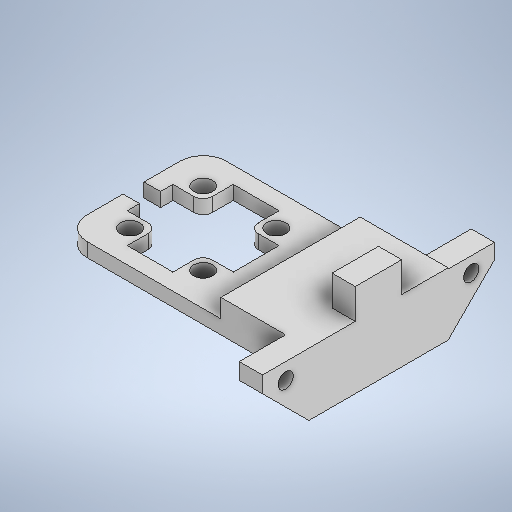
# Autodesk Inventor part: as5600mount
Saved by Autodesk Inventor 2025.2 (Build 292293000, 293)
## iProperties
Created: 2024-11-28
Part Number: as5600mount
Material: Generic
Document SubType Name: Modeling
Designer: email
Density: 1 g/cm^3
Appearance: Default
Author: email
Autodesk Inventor part; units mm, degrees
ref_plane "YZ Plane" through (0, 0, 0) normal (1, 0, 0) x (0, 1, 0)
ref_plane "XZ Plane" through (0, 0, 0) normal (0, 1, 0) x (-1, 0, 0)
ref_plane "XY Plane" through (0, 0, 0) normal (0, 0, 1) x (1, 0, 0)
sketch "Sketch1" plane through (0, 0, 0) normal (0, 1, 0) x (-1, 0, 0)
  line L0 (0, 0) -> (-22.86, 0)
  line L1 (-22.86, 0) -> (-22.86, -22.86)
  line L2 (-22.86, -22.86) -> (0, -22.86)
  line L3 (0, -22.86) -> (0, 0)
  line L4 (-22.86, -22.86) -> (-19.304, -22.86)
  line L5 (-19.304, -22.86) -> (-19.304, -19.304) construction
  line L6 (-19.304, -19.304) -> (-22.86, -19.304) construction
  line L7 (-22.86, -19.304) -> (-22.86, -22.86)
  line L8 (0, -22.86) -> (-3.556, -22.86)
  line L9 (-3.556, -22.86) -> (-3.556, -19.304) construction
  line L10 (-3.556, -19.304) -> (0, -19.304) construction
  line L11 (0, -19.304) -> (0, -22.86)
  line L12 (0, 0) -> (-3.556, 0)
  line L13 (-3.556, 0) -> (-3.556, -3.556) construction
  line L14 (-3.556, -3.556) -> (0, -3.556) construction
  line L15 (0, -3.556) -> (0, 0)
  line L16 (-22.86, 0) -> (-19.304, 0)
  line L17 (-19.304, 0) -> (-19.304, -3.556) construction
  line L18 (-19.304, -3.556) -> (-22.86, -3.556) construction
  line L19 (-22.86, -3.556) -> (-22.86, 0)
  circle A0 centre (-3.556, -19.304) radius 2.075
  circle A1 centre (-19.304, -19.304) radius 2.075
  circle A2 centre (-19.304, -3.556) radius 2.075
  circle A3 centre (-3.556, -3.556) radius 2.075
  line L20 (3.57, -26.43) -> (-26.43, -26.43)
  line L21 (-26.43, -26.43) -> (-26.43, 3.57)
  line L22 (-26.43, 3.57) -> (3.57, 3.57)
  line L23 (3.57, 3.57) -> (3.57, -26.43)
  line L24 (0, 0) -> (-6.5, 0)
  line L25 (-6.5, 0) -> (-6.5, -6.5)
  line L26 (-6.5, -6.5) -> (0, -6.5)
  line L27 (0, -6.5) -> (0, 0)
  line L28 (0, -22.86) -> (-6.5, -22.86)
  line L29 (-6.5, -22.86) -> (-6.5, -16.36)
  line L30 (-6.5, -16.36) -> (0, -16.36)
  line L31 (0, -16.36) -> (0, -22.86)
  line L32 (-22.86, -22.86) -> (-16.36, -22.86)
  line L33 (-16.36, -22.86) -> (-16.36, -16.36)
  line L34 (-16.36, -16.36) -> (-22.86, -16.36)
  line L35 (-22.86, -16.36) -> (-22.86, -22.86)
  line L36 (-22.86, 0) -> (-16.36, 0)
  line L37 (-16.36, 0) -> (-16.36, -6.5)
  line L38 (-16.36, -6.5) -> (-22.86, -6.5)
  line L39 (-22.86, -6.5) -> (-22.86, 0)
  line L40 (-26.43, 3.57) -> (-49.205, 3.57)
  line L41 (-49.205, 3.57) -> (-49.205, -26.43)
  line L42 (-49.205, -26.43) -> (-26.43, -26.43)
  line L43 (-26.43, -26.43) -> (-26.43, 3.57)
  circle A4 centre (-11.43, -11.43) radius 5
  line L44 (-9.3887, -15.2384) -> (-13.3887, -15.2384)
  line L45 (-13.3887, -15.2384) -> (-13.3887, -23.9816)
  line L46 (-13.3887, -23.9816) -> (-9.3887, -23.9816)
  line L47 (-9.3887, -15.2384) -> (-13.3887, -23.9816) construction
  line L48 (-13.3887, -15.2384) -> (-9.3887, -23.9816) construction
  line L49 (5.2257, -13.68) -> (-9.4126, -13.68)
  line L50 (-9.4126, -13.68) -> (-9.4126, -9.18)
  line L51 (-9.4126, -9.18) -> (5.2257, -9.18)
  line L52 (5.2257, -9.18) -> (5.2257, -13.68)
  line L53 (5.2257, -13.68) -> (-9.4126, -9.18) construction
  line L54 (-9.4126, -13.68) -> (5.2257, -9.18) construction
  point P0 (0, -16.36)
  point P1 (0, -6.5)
  point P2 (-11.3887, -19.61)
  point P3 (-2.0935, -11.43)
  point P4 (0, -9.18)
  point P5 (3.57, -9.18)
  point P6 (3.57, -13.68)
  point P7 (0, -13.68)
  dimension "d2" = 22.86
  dimension "d3" = 22.86
  dimension "d4" = 3.556
  dimension "d5" = 3.556
  dimension "d6" = 3.556
  dimension "d7" = 3.556
  dimension "d8" = 3.556
  dimension "d9" = 3.556
  dimension "d10" = 3.556
  dimension "d11" = 3.556
  dimension "d12" = 4.15
  dimension "d13" = 4.15
  dimension "d14" = 4.15
  dimension "d15" = 4.15
  dimension "d16" = 30
  dimension "d17" = 30
  dimension "d18" = 3.57
  dimension "d19" = 3.57
  dimension "d20" = 6.5
  dimension "d21" = 6.5
  dimension "d22" = 6.5
  dimension "d23" = 6.5
  dimension "d24" = 6.5
  dimension "d25" = 6.5
  dimension "d26" = 6.5
  dimension "d31" = 10
  dimension "d32" = 15
  dimension "d33" = 15
  dimension "d34" = 37.775
  dimension "d69" = 4
  dimension "d70" = 4.5
  constraints: 110 end point, 25 parallel, 13 horizontal, 13 perpendicular, 5 centre point, 4 coincident, 4 midpoint, 2 point on line
  measures "d2" distance of L4.start L3.start
  measures "d3" distance of L0.end L4.start
  measures "d4" distance of L9.start L9.end
  measures "d5" distance of L9.end L11.start
  measures "d6" distance of L13.end L15.start
  measures "d7" distance of L13.start L13.end
  measures "d8" distance of L18.start L18.end
  measures "d9" distance of L17.start L18.start
  measures "d10" distance of L5.end L7.start
  measures "d11" distance of L5.start L5.end
  measures "d12" diameter of A0
  measures "d13" diameter of A1
  measures "d14" diameter of A2
  measures "d15" diameter of A3
  measures "d16" distance of L20.start L20.end
  measures "d17" distance of L20.end L21.end
  measures "d18" distance between parallel lines of L3 L23
  measures "d19" distance between parallel lines of L2 L20
  measures "d20" distance of L25.end L26.end
  measures "d21" distance of L24.end L25.end
  measures "d22" distance of L28.end L29.end
  measures "d23" distance of L29.end L30.end
  measures "d24" distance of L32.end L33.end
  measures "d25" distance of L33.end L34.end
  measures "d26" distance of L36.end L37.end
  measures "d31" diameter of A4
  measures "d32" distance from line of L20 A4.centre
  measures "d33" distance from line of L23 A4.centre
  measures "d34" distance from line of L41 A4.centre
  measures "d69" distance of L45.end L46.end
  measures "d70" distance between parallel lines of L49 L51
extrude "Extrusion1" add sketch "Sketch1" along normal blind 7 contours L3 L26 L25 L0 | L0 L1 L2 L3 L49 L23 L20 L21 L22 L51 | L37 L38 L1 L0 | L3 L2 L29 L30 | L34 L33 L2 L1 | L21 L42 L41 L40
fillet "Fillet1" radius 2 4 edges at (6.5, 3.5, -16.36) (16.36, 3.5, -16.36) (16.36, 3.5, -6.5) (6.5, 3.5, -6.5)
sketch "Sketch4" plane through (49.205, 0, 3.57) normal (1, 0, 0) x (0, 0, -1)
  line L0 (-10, 13.5061) -> (40, 13.5061)
  line L1 (40, 13.5061) -> (40, -6.4939)
  line L2 (40, -6.4939) -> (-10, -6.4939)
  line L3 (-10, -6.4939) -> (-10, 13.5061)
  line L4 (-10, 13.5061) -> (40, -6.4939) construction
  line L5 (40, 13.5061) -> (-10, -6.4939) construction
  line L6 (30, 0) -> (30, 7) projected
  line L7 (15, 3.5061) -> (35, 3.5061)
  circle A0 centre (35, 3.5061) radius 1.65
  circle A1 centre (-5, 3.5061) radius 1.65
  line L8 (-10, 0) -> (40, 0)
  line L9 (40, 0) -> (40, 13.5061)
  line L10 (40, 13.5061) -> (-10, 13.5061)
  line L11 (-10, 13.5061) -> (-10, 0)
  line L12 (-10, -6.4939) -> (0, -6.4939)
  line L13 (0, -6.4939) -> (0, 0)
  line L14 (0, 0) -> (-10, 0)
  line L15 (-10, 0) -> (-10, -6.4939)
  line L16 (40, -6.4939) -> (30, -6.4939)
  line L17 (30, -6.4939) -> (30, 0)
  line L18 (30, 0) -> (40, 0)
  line L19 (40, 0) -> (40, -6.4939)
  line L20 (40, 13.5061) -> (20, 13.5061)
  line L21 (20, 13.5061) -> (20, 6.753)
  line L22 (20, 6.753) -> (40, 6.753)
  line L23 (40, 6.753) -> (40, 13.5061)
  line L24 (0, 7) -> (30, 7) projected
  line L25 (-10, 13.5061) -> (10, 13.5061)
  line L26 (10, 13.5061) -> (10, 7)
  line L27 (10, 7) -> (-10, 7)
  line L28 (-10, 7) -> (-10, 13.5061)
  point P0 (3.57, 0)
  point P1 (40, -3.247)
  point P2 (-10, -3.247)
  point P3 (-10, 10.253)
  point P4 (10, 10.253)
  point P5 (40, 10.1296)
  point P6 (20, 13.5061)
  point P7 (10, 13.5061)
  point P8 (-10, 7)
  point P9 (40, 6.753)
  dimension "d46" = 50
  dimension "d47" = 20
  dimension "d48" = 15
  dimension "d49" = 10
  dimension "d56" = 20
  dimension "d57" = 20
  dimension "d58" = 3.3
  dimension "d59" = 3.3
  dimension "d66" = 10
  dimension "d67" = 20
  dimension "d68" = 20
  constraints: 54 end point, 12 parallel, 7 horizontal, 7 midpoint, 6 perpendicular, 3 point on line, 2 centre point, 1 coincident
  measures "d46" distance of L1.end L2.end
  measures "d47" distance of L0.end L1.end
  measures "d48" distance from line of L6 L7.start
  measures "d49" distance from line of L7.start L2
  measures "d56" distance of L7.start L7.end
  measures "d57" distance of L7.start A1.centre
  measures "d58" diameter of A0
  measures "d59" diameter of A1
  measures "d66" distance from line of L13 point (-10, -3.247)
  measures "d67" distance of point (-10, 10.253) point (10, 10.253)
  measures "d68" distance from line of point (40, 10.13) L21
extrude "Extrusion4" add sketch "Sketch4" against normal blind 5 contours L0 L21 L24 L26 | L27 L24 L21 L22 L6 L8 L3 | L8 L13 L2 L3 | L8 L17 L2 L13 | L1 L8 L6 L22 | L8 L1 L2 L17
fillet "Fillet2" radius 5 2 edges at (-3.57, 3.5, -26.43) (-3.57, 3.5, 3.57)
chamfer "Chamfer1" distance 10 angle 45 2 edges at (46.705, -6.4939, 13.57) (46.705, -6.4939, -36.43)
sketch "Sketch5" plane through (0, 7, 0) normal (0, 1, 0) x (1, 0, 0)
  line L0 (-8.8762, -11.5964) -> (30.2556, -11.5964)
  line L1 (30.2556, -11.5964) -> (30.2556, 37.6524)
  line L2 (30.2556, 37.6524) -> (-8.8762, 37.6524)
  line L3 (-8.8762, 37.6524) -> (-8.8762, -11.5964)
  point P0 (0, 0)
  constraints: 8 end point, 2 parallel, 1 horizontal, 1 perpendicular
extrude "Extrusion5" cut sketch "Sketch5" against normal blind 4
body "Solid1"
